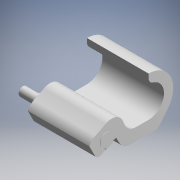
# Autodesk Inventor part: CE2-M9P_BA7-063(63)_2
Saved by Autodesk Inventor 2017.3 (Build 213256000, 256)
## iProperties
Part Number: CE2-M9P_BA7-063(63)_2
Material: Generic
Catalog Web Link: www.cadenas.de
Description: CE2 AUTOSWITCH2-Stroke Reading Cylinder with Brake
Vendor: SMC
Document SubType Name: Modeling
Designer: partserver
Manufacturer: SMC
Mass: 3.46326 g
Surface Area: 23.4673 cm^2
Volume: 3.46326 cm^3
Density: 1 g/cm^3
Appearance: PSOLRGB-255-255-255
Category: PARTsolutions
Company: SMC
Title: CE2-M9P_BA7-063(63)
Author: Cadenas PARTsolutions
Comments: Stroke Reading Cylinder with Brake
PSOL_IDENT_0: {$CADENAS_DATA\23d-libs\smc_jp\actuator\stroke_reading_cylinders\ce2\parts\ce2_asw2.prj},200 {VTYP=3
PSOL_IDENT_1: D},{NB=CE2-M9P_BA7-063(63)_2},{LINA=CE2-M9P_BA7-063(63)},{NN=CE2 AUTOSWITCH2},{DATE=05.07.2021 01:49
PSOL_IDENT_2: :15},{GEOMDATE=05.03.2012 09:14:00},{VERSION=},{LINEID=80},{WBVAR=AUTOSWITCH1},{WBNUMERIC=}  {NB=CE2
PSOL_IDENT_3: -M9P_BA7-063(63)_2},{LINA=CE2-M9P_BA7-063(63)},{KT=DUMMY},{ORDER=CE2-M9P_BA7-063(63)},{OUTD0=68.000}
PSOL_IDENT_4: ,{OUTD=72},{BORE=63},{AUTOSWITCH1=-M9P},{AUTOSWX='','(-) Without autoswitch (Built-in magnet)','-M9N'
PSOL_IDENT_5: ,'M9N','-M9P','M9P','-M9B','M9B','-J51','J51','-G39C','G39C','-K39C','K39C','-M9NW','M9NW','-M9PW','
PSOL_IDENT_6: M9PW','-M9BW','M9BW','-M9NA','M9NA','-M9PA','M9PA','-M9BA','M9BA','-F59F','F59F','-A96','A96','-A93'
PSOL_IDENT_7: ,'A93','-A90','A90','-A54','A54','-A64','A64','-A33C','A33C','-A34C','A34C','-A44C','A44C','-A59W','
PSOL_IDENT_8: A59W','-G59','G59','-G5P','G5P','-K59','K59','-G39','G39','-K39','K39','-G59W','G59W','-G5PW','G5PW'
PSOL_IDENT_9: ,'-K59W','K59W','-G5BA','G5BA','-G59F','G59F','-B54','B54','-B64','B64','-A33','A33','-A34','A34','-
PSOL_IDENT_10: A44','A44','-B59W','B59W'},{SWITCHS=J},{SWMOUNT=BA7-063},{SWHS1=0.7},{B=85},{C=64},{JN=10},{J2=10.5}
PSOL_IDENT_11: ,{A33HS=85.0},{A33HS2=4.0},{A33CHS=85.5},{A33CHS2=4.5},{A44HS=93.5},{A44HS2=3.7},{A44CHS=93.5},{A44C
PSOL_IDENT_12: HS2=3.8},{F59HS=47.0},{A53HS=46.5},{Y59AHS=41.0},{Y69AHS=41.0},{P4DWLHS=52.0},{P4DWLHT=43.0},{M9NHS=
PSOL_IDENT_13: 41.0},{M9NVHS=44.0},{A90VHS=41.5},{HW=91},{H=61.5},{H2=53.0},{T=10.5},{T2=7.5},{H3=60.5},{H4=52.0},{
PSOL_IDENT_14: A1=8.5},{B1=7.5},{A2=12.5},{B2=11.5},{A3=6.0},{B3=5.0},{A4=5.5},{B4=4.5},{A5=2.5},{B5=1.5},{A6=3.0},
PSOL_IDENT_15: {B6=2.0},{A7=9.0},{B7=8.0},{A8=4.5},{B8=3.5},{A9=6.5},{B9=5.5},{A10=14.0},{B10=13.0},{AUTOSWITCH=M9P
PSOL_IDENT_16: }
NB: CE2-M9P_BA7-063(63)_2
NN: CE2 AUTOSWITCH2
NT: Stroke Reading Cylinder with Brake
NBSYN: $ORDER._2
LINA: CE2-M9P_BA7-063(63)
CATALOG: SMC (JP
OUTD0: 68
OUTD: 72
BORE: 63
AUTOSWITCH1: M9P
SWHS1: 0.7
B: 85
C: 64
JN: 10
J2: 10.5
A33HS: 85
A33HS2: 4
A33CHS: 85.5
A33CHS2: 4.5
A44HS: 93.5
A44HS2: 3.7
A44CHS: 93.5
A44CHS2: 3.8
F59HS: 47
A53HS: 46.5
Y59AHS: 41
Y69AHS: 41
P4DWLHS: 52
P4DWLHT: 43
M9NHS: 41
M9NVHS: 44
A90VHS: 41.5
HW: 91
H: 61.5
H2: 53
T: 10.5
T2: 7.5
H3: 60.5
H4: 52
A1: 8.5
B1: 7.5
A2: 12.5
B2: 11.5
A3: 6
B3: 5
A4: 5.5
B4: 4.5
A5: 2.5
B5: 1.5
A6: 3
B6: 2
A7: 9
B7: 8
A8: 4.5
B8: 3.5
A9: 6.5
B9: 5.5
A10: 14
B10: 13
SUPPLIER: SMC
ARTICLENO: CE2-M9P_BA7-063(63)_2
BOMINFO: CE2-M9P_BA7-063(63)
CREATOR: CADENAS GmbH
Autodesk Inventor part; units mm, degrees
sketch "Sketch_1" plane through (0, 0, 0) normal (1, 0, 0) x (0, 1, 0)
  line L0 (34.0472, 41) -> (26.1009, 41)
  arc A0 (26.1009, 41) -> (22.5392, 38.8206) centre (26.1009, 37) ccw
  line L1 (22.5392, 38.8206) -> (21.4582, 36.7057)
  line L2 (21.4582, 36.7057) -> (21.013, 36.9333)
  arc A1 (21.013, 36.9333) -> (20.3402, 36.7156) centre (20.7854, 36.4881) ccw
  line L3 (20.3402, 36.7156) -> (20.08, 36.2066)
  arc A2 (17.5868, 37.481) -> (20.08, 36.2066) centre (18.1833, 35.572) ccw
  line L4 (17.5868, 37.481) -> (17.847, 37.9901)
  arc A3 (17.847, 37.9901) -> (17.6294, 38.6628) centre (17.4018, 38.2176) ccw
  line L5 (17.6294, 38.6628) -> (16.6499, 39.1635)
  arc A4 (16.6499, 39.1635) -> (14.6316, 38.5106) centre (15.9672, 37.8279) ccw
  line L6 (14.6316, 38.5106) -> (12.7552, 34.8399)
  arc A5 (12.7552, 34.8399) -> (14.7622, 32.8341) centre (16.4025, 36.4823) ccw
  arc A6 (17.9677, 31.1955) -> (14.7622, 32.8341) centre (0, 0) ccw
  arc A7 (17.9677, 31.1955) -> (23.6461, 33.0988) centre (19.9641, 34.6617) ccw
  line L7 (23.6461, 33.0988) -> (24.2676, 34.5629)
  arc A8 (27.9496, 37) -> (24.2676, 34.5629) centre (27.9496, 33) ccw
  line L8 (27.9496, 37) -> (32, 37)
  arc A9 (33.4286, 27.2084) -> (32, 37) centre (32, 32) ccw
  arc A10 (33.4286, 27.2084) -> (32, 25.2918) centre (34, 25.2918) ccw
  line L9 (32, 25.2918) -> (32, 24)
  arc A11 (32, 24) -> (38.2125, 37.0403) centre (32, 32) ccw
  line L10 (38.2125, 37.0403) -> (35.6003, 40.2601)
  arc A12 (35.6003, 40.2601) -> (34.0472, 41) centre (34.0472, 39) ccw
  constraints: 26 point on circle, 22 end point, 13 centre point
extrude "Extrusion1" add sketch "Sketch_1" along normal blind 20.1
sketch "Sketch_2" plane through (0, 0, 0) normal (0, 0, 1) x (1, 0, 0)
  line L0 (0, 42.5) -> (0, -42.5)
  line L1 (0, -42.5) -> (0.1, -42.5)
  line L2 (0.1, -42.5) -> (0.1, 42.5)
  line L3 (0.1, 42.5) -> (0, 42.5)
  constraints: 8 end point
extrude "Extrusion2" cut sketch "Sketch_2" along normal mid plane 200
sketch "Sketch3" plane through (20.1, 26.1009, 41) normal (0, 0, 1) x (1, 0, 0)
  point P0 (-4, 5.7463)
hole "Hole1" at (16.1, 31.8472, 41) direction (0, 0, -1) diameter 4 depth 0.5
pattern_linear "Rectangular Pattern1" count 2 spacing 12 along (-1, 0, 0) of "Hole1"
sketch "Sketch_5" plane through (16.1, 31.8472, 40.5) normal (0, 0, 1) x (0, -1, 0)
  line L0 (-1.25, -0.7217) -> (0, -1.4434)
  line L1 (0, -1.4434) -> (1.25, -0.7217)
  line L2 (1.25, -0.7217) -> (1.25, 0.7217)
  line L3 (1.25, 0.7217) -> (0, 1.4434)
  line L4 (0, 1.4434) -> (-1.25, 0.7217)
  line L5 (-1.25, 0.7217) -> (-1.25, -0.7217)
  constraints: 12 end point
extrude "Extrusion3" cut sketch "Sketch_5" against normal blind 1
pattern_linear "Rectangular Pattern2" count 2 spacing 12 along (-1, 0, 0) of "Extrusion3"
sketch "Sketch_7" plane through (0, 0, 0) normal (1, 0, 0) x (0, 1, 0)
  line L0 (18.1201, 38.5243) -> (17.5868, 37.481)
  arc A0 (17.5868, 37.481) -> (20.08, 36.2066) centre (18.1833, 35.572) ccw
  line L1 (20.08, 36.2066) -> (20.6133, 37.2499)
  line L2 (20.6133, 37.2499) -> (18.1201, 38.5243)
  constraints: 6 end point, 2 point on circle, 1 centre point
extrude "Extrusion4" add sketch "Sketch_7" along normal blind 22
sketch "Sketch_8" plane through (0, 0, 0) normal (1, 0, 0) x (0, 1, 0)
  arc A0 (19.4991, 35.1802) -> (17.095, 36.4091) centre (18.2971, 35.7946) ccw
  line L0 (17.095, 36.4091) -> (16.8674, 35.9639)
  arc A1 (16.8674, 35.9639) -> (19.2716, 34.735) centre (18.0695, 35.3494) ccw
  line L1 (19.2716, 34.735) -> (19.4991, 35.1802)
  constraints: 4 end point, 4 point on circle, 2 centre point
extrude "Extrusion5" add sketch "Sketch_8" along normal blind 27
sketch "Sketch_9" plane through (0, 20.6133, 37.2499) normal (0, 0.4551514, 0.890414) x (1, 0, 0)
  circle A0 centre (2, -1.4) radius 1.25
  circle A1 centre (2, -1.4) radius 1.05
  constraints: 2 centre point
extrude "Extrusion6" cut sketch "Sketch_9" against normal blind 1
sketch "Sketch_10" plane through (0, 20.6133, 37.2499) normal (0, 0.4551514, 0.890414) x (1, 0, 0)
  arc A0 (0.9663, -2.0095) -> (1.3905, -2.4337) centre (2, -1.4) ccw
  line L0 (1.3905, -2.4337) -> (3.0337, -0.7905)
  arc A1 (3.0337, -0.7905) -> (2.6095, -0.3663) centre (2, -1.4) ccw
  line L1 (2.6095, -0.3663) -> (0.9663, -2.0095)
  constraints: 4 end point, 4 point on circle, 2 centre point
extrude "Extrusion7" cut sketch "Sketch_10" against normal blind 0.5
sketch "Sketch_11" plane through (0, 20.6133, 37.2499) normal (0, 0.4551514, 0.890414) x (1, 0, 0)
  arc A0 (8, -1.8) -> (8.4, -2.2) centre (8.4, -1.8) ccw
  line L0 (8.4, -2.2) -> (10.6, -2.2)
  arc A1 (10.6, -2.2) -> (11, -1.8) centre (10.6, -1.8) ccw
  line L1 (11, -1.8) -> (11, -1)
  arc A2 (11, -1) -> (10.6, -0.6) centre (10.6, -1) ccw
  line L2 (10.6, -0.6) -> (8.4, -0.6)
  arc A3 (8.4, -0.6) -> (8, -1) centre (8.4, -1) ccw
  line L3 (8, -1) -> (8, -1.8)
  constraints: 8 end point, 8 point on circle, 4 centre point
extrude "Extrusion8" cut sketch "Sketch_11" against normal blind 0.2
ref_plane "sw_XY" through (-11.5, 0, 0) normal (1, 0, 0) x (0, 0, -1)
ref_plane "sw_YZ" through (-11.5, 0, 0) normal (0, 0, -1) x (0, 1, 0)
ref_plane "sw_ZX" through (-11.5, 0, 0) normal (0, 1, 0) x (1, 0, 0)
body "Solid1"
